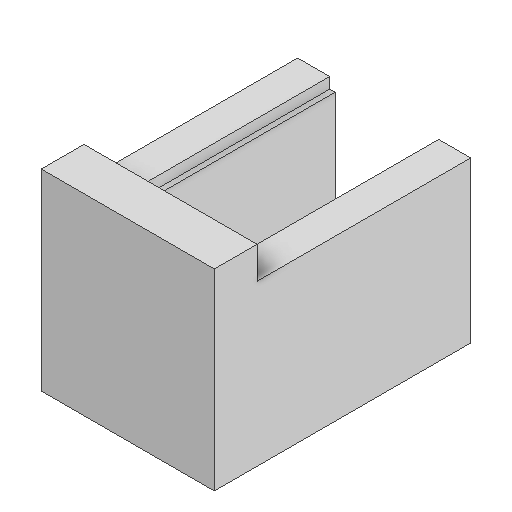
# Autodesk Inventor part: 30_XY_Sample_lightsheetarm_sample_box
Saved by Autodesk Inventor 2022 (Build 260153000, 153)
## iProperties
Created: 2021-11-10
Part Number: 30_XY_Sample_lightsheetarm_sample_box
Material: Generic
Document SubType Name: Modeling
Designer: diederichbenedict
Density: 1 g/cm^3
Appearance: Default
Author: diederichbenedict
Autodesk Inventor part; units mm, degrees
ref_plane "YZ Plane" through (0, 0, 0) normal (1, 0, 0) x (0, 1, 0)
ref_plane "XZ Plane" through (0, 0, 0) normal (0, 1, 0) x (-1, 0, 0)
sketch "Sketch1" plane through (0, 0, 0) normal (0, 0, 1) x (1, 0, 0)
  line L0 (0, 4) -> (0, -2) projected
  line L1 (0, 4) -> (-10, 4) projected
  line L2 (-10, 1.0237) -> (-13, 1.0237)
  line L3 (-13, 1.0237) -> (-13, -13.9763)
  line L4 (-13, -13.9763) -> (-10, -13.9763)
  line L5 (-10, -13.9763) -> (-10, 1.0237)
  line L6 (0.2, 1.0237) -> (3.2, 1.0237)
  line L7 (3.2, 1.0237) -> (3.2, -13.9763)
  line L8 (3.2, -13.9763) -> (0.2, -13.9763)
  line L9 (0.2, -13.9763) -> (0.2, 1.0237)
  line L10 (-10, 0) -> (-9.5, 0)
  line L11 (-9.5, 0) -> (-9.5, -13.9763)
  line L12 (-9.5, -13.9763) -> (-10, -13.9763)
  line L13 (-10, -13.9763) -> (-10, 0)
  line L14 (0.2, -13.9763) -> (-0.3, -13.9763)
  line L15 (-0.3, -13.9763) -> (-0.3, 0)
  line L16 (-0.3, 1.0237) -> (0, 1.0237)
  line L17 (0.2, 1.0237) -> (0.2, -13.9763)
  line L18 (-0.3, 0) -> (0.2, 0)
  line L19 (-10, -2) -> (-10, 4) projected
  line L20 (0, -2) -> (-10, -2) projected
  dimension "d0" = 3
  dimension "d1" = 15
  dimension "d2" = 3
  dimension "d3" = 0.2
  dimension "d6" = 0.5
  dimension "d7" = 0.5
  constraints: 34 end point, 8 parallel, 5 perpendicular, 4 horizontal, 4 point on line
  measures "d0" distance of L4.end L3.end
  measures "d1" distance of L3.end L2.end
  measures "d2" distance of L7.end L8.end
  measures "d3" distance between parallel lines of L0 L9
  measures "d6" distance of L11.end L12.end
  measures "d7" distance of L16.start L17.start
ref_plane "Work Plane1" through (-32, -64, -20) normal (0, 0, -1) x (0, 1, 0)
extrude "Extrusion1" add sketch "Sketch1" against normal up to surface (20 mm away) contours L18 L9 L14 L15 L20 L0 | L0 L20 L15 L18 | L5 L4 L3 L2 | L9 L6 L7 L8 | L10 L11 L20 L5 | L20 L11 L12 L5
sketch "Sketch2" plane through (0, 0, 0) normal (0, 0, 1) x (1, 0, 0)
  line L0 (-10, 0) -> (-10, 1.0237) projected
  line L1 (-10, 1.0237) -> (-13, 1.0237) projected
  line L2 (-13, 1.0237) -> (-13, -13.9763) projected
  line L3 (-13, -13.9763) -> (-9.5, -13.9763) projected
  line L4 (-9.5, -13.9763) -> (-9.5, 0) projected
  line L5 (-9.5, 0) -> (-10, 0) projected
  line L6 (3.2, -13.9763) -> (3.2, 1.0237) projected
  line L7 (-13, 1.0237) -> (-13, -13.9763) projected
  line L8 (-13, -13.9763) -> (3.2, -13.9763)
  line L9 (3.2, -13.9763) -> (3.2, 4.022)
  line L10 (3.2, 4.022) -> (-13, 4.022)
  line L11 (-13, 4.022) -> (-13, -13.9763)
  line L12 (3.2, 1.0237) -> (0.2, 1.0237) projected
  line L13 (0.2, 1.0237) -> (0.2, 0) projected
  line L14 (-0.3, -13.9763) -> (3.2, -13.9763) projected
  line L15 (0.2, 0) -> (-0.3, 0) projected
  line L16 (-0.3, 0) -> (-0.3, -13.9763) projected
  point P0 (0, 0)
  point P1 (0.2, -13.9763)
  constraints: 8 end point, 2 parallel, 1 horizontal, 1 perpendicular
extrude "Extrusion2" add sketch "Sketch2" along normal blind 4
sketch "Sketch3" plane through (-0.3, -13.9763, -20) normal (0, -1, 0) x (1, 0, 0)
  line L0 (0, 0) -> (3.5, 0) projected
  line L1 (3.5, 0) -> (3.5, 24) projected
  line L2 (-12.7, 24) -> (3.5, 24) projected
  line L3 (-12.7, 0) -> (-12.7, 24) projected
  line L4 (-12.7, 0) -> (-9.2, 0) projected
  line L5 (-9.2, 20) -> (-9.2, 0) projected
  line L6 (0.3, 4) -> (-9.7, 4) projected
  line L7 (-9.2, 20) -> (-9.2, 0) projected
  line L8 (0, 20) -> (0, 0) projected
  line L9 (-9.2, 4) -> (0, 4)
  line L10 (0, 4) -> (0, 6)
  line L11 (0, 6) -> (-9.2, 6)
  line L12 (-9.2, 6) -> (-9.2, 4)
  line L13 (-9.2, 20) -> (0.3, 20)
  line L14 (0.3, 20) -> (0.3, 18)
  line L15 (0.3, 18) -> (-9.2, 18)
  line L16 (-9.2, 18) -> (-9.2, 20)
  line L17 (-9.2, 20) -> (0, 20) projected
  line L18 (0, 20) -> (0, 0) projected
  point P0 (0.3, 20)
  dimension "d10" = 2
  dimension "d11" = 2
  constraints: 16 end point, 4 parallel, 3 point on line, 2 horizontal, 2 perpendicular
  measures "d10" distance of L10.end L9.end
  measures "d11" distance of L13.end L14.end
extrude "Extrusion3" [suppressed]
body "Solid1"
